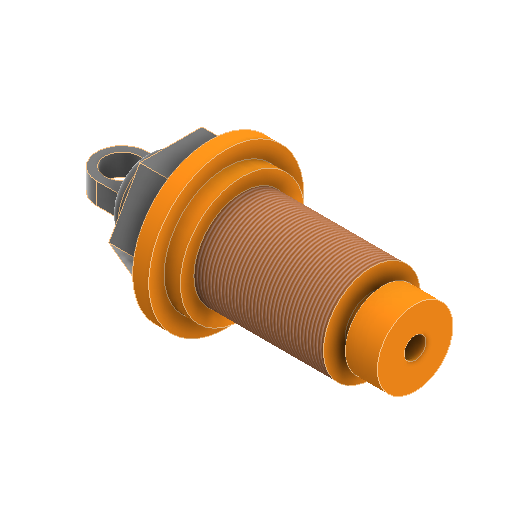
# Autodesk Inventor part: 100MMshockUpper
Saved by Autodesk Inventor 2025 (Build 290162000, 162)
## iProperties
Created: 2024-10-22
Part Number: 100MMshockUpper
Material: Generic
Document SubType Name: Modeling
Designer: derm
Density: 1 g/cm^3
Appearance: Orange
Author: derm
Autodesk Inventor part; units mm, degrees
ref_plane "YZ Plane" through (0, 0, 0) normal (1, 0, 0) x (0, 1, 0)
ref_plane "XZ Plane" through (0, 0, 0) normal (0, 1, 0) x (-1, 0, 0)
ref_plane "XY Plane" through (0, 0, 0) normal (0, 0, 1) x (1, 0, 0)
sketch "Sketch1" plane through (0, 0, 0) normal (0, 1, 0) x (-1, 0, 0)
  line L0 (0, 0) -> (50, 0)
  line L1 (0, 0) -> (0, -7)
  line L2 (0, -7) -> (6, -7)
  line L3 (6, -7) -> (6, -5)
  line L4 (6, -5) -> (8, -5)
  line L5 (8, -5) -> (8, -9)
  line L6 (8, -9) -> (32, -9)
  line L7 (32, -9) -> (32, -11.5)
  line L8 (32, -11.5) -> (35, -11.5)
  line L9 (35, -11.5) -> (35, -14.3615)
  line L10 (35, -14.3615) -> (38, -14.3615)
  line L11 (38, -14.3615) -> (38, -11.5)
  line L12 (38, -11.5) -> (45.2698, -11.5)
  line L13 (45.2698, -11.5) -> (45.2698, -7)
  line L14 (45.2698, -7) -> (50, -7)
  line L15 (50, -7) -> (50, 0)
  line L16 (0, 0) -> (27.4762, 0)
  line L17 (27.4762, 0) -> (27.4762, -2)
  line L18 (27.4762, -2) -> (0, -2)
  line L19 (0, -2) -> (0, 0)
  point P0 (7, -5)
  point P1 (32, -10.25)
  dimension "d0" = 50
  dimension "d1" = 7
  dimension "d2" = 6
  dimension "d3" = 2
  dimension "d4" = 5
  dimension "d6" = 24
  dimension "d7" = 3
  dimension "d8" = 3
  dimension "d9" = 11.5
  dimension "d10" = 9
  dimension "d12" = 2
  constraints: 40 end point, 12 perpendicular, 4 point on line, 2 horizontal, 2 midpoint, 2 parallel, 1 vertical
  measures "d0" distance of L0.start L0.end
  measures "d1" distance of L0.start L1.end
  measures "d2" distance of L1.end L2.end
  measures "d3" distance of L3.end L4.end
  measures "d4" distance from line of point (7, -5) L0
  measures "d6" distance from line of L5 point (32, -10.25)
  measures "d7" distance of L7.end L8.end
  measures "d8" distance of L9.end L10.end
  measures "d9" distance between parallel lines of L0 L12
  measures "d10" distance between parallel lines of L0 L6
  measures "d12" distance of L16.end L17.end
revolve "Revolution1" add sketch "Sketch1" angle 360 about axis through (0, 0, 0) along (-1, 0, 0) contours L0 L15 L14 L13 L12 L11 L10 L9 L8 L7 L6 L5 L4 L3 L2 L1 L18 L17
sketch "Sketch2" plane through (0, 0, 0) normal (0, 1, 0) x (-1, 0, 0)
  line L0 (50, -7) -> (50, 7) projected
  line L1 (45.2698, -7) -> (45.2698, 7) projected
  circle A0 centre (54.2556, 0) radius 3.25
  arc A1 (54.2556, -4.7218) -> (54.2556, 4.7218) centre (54.2556, 0) ccw
  line L2 (54.2556, 4.7218) -> (50, 4.7218)
  line L3 (54.2556, -4.7218) -> (50, -4.7218)
  point P0 (0, 0)
  dimension "d13" = 6.5
  constraints: 4 end point, 2 centre point, 2 perpendicular, 2 point on circle, 2 point on line, 2 tangent, 1 coincident
  measures "d13" diameter of A0
extrude "Extrusion1" add sketch "Sketch2" along normal mid plane 4
fillet "Fillet1" radius 2 1 edges at (-50, 0, 7)
sketch "Sketch3" plane through (-45.2698, 0, 0) normal (-1, 0, 0) x (0, 0, 1)
  circle A0 centre (0, 0) radius 11.5 projected
  circle A1 centre (0, 0) radius 2 projected
  line L0 (11.5, 0) -> (5.75, -9.9593)
  line L1 (5.75, -9.9593) -> (-5.75, -9.9593)
  line L2 (-5.75, -9.9593) -> (-11.5, 0)
  line L3 (-11.5, 0) -> (-5.75, 9.9593)
  line L4 (-5.75, 9.9593) -> (5.75, 9.9593)
  line L5 (5.75, 9.9593) -> (11.5, 0)
  point P0 (-11.5, 0)
  point P1 (-11.5, 0)
  point P2 (-5.75, -9.9593)
  point P3 (-5.75, -9.9593)
  constraints: 12 end point, 1 coincident, 15 other
extrude "Extrusion2" cut sketch "Sketch3" against normal up to surface (7.2698 mm away) contours L5 A0 | A0 L0 | L4 A0 | A0 L1 | L3 A0 | A0 L2
thread "Thread1" size "5-40 UNC" class "2A" standard "ANSI Unified Screw Threads" full length
body "Solid1"
